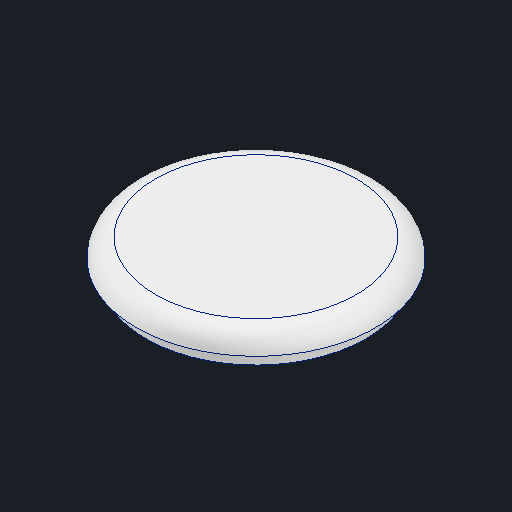
# Autodesk Inventor part: Tapa
Saved by Autodesk Inventor 2025.3 (Build 293356030, 356C)
## iProperties
Created: 2024-12-23
Part Number: Tapa
Material: Aluminio 6061
Document SubType Name: Modeling
Designer: Usuario
Density: 2.7 g/cm^3
Appearance: Aluminio - Plano
Mass: 96.7212 g
Surface Area: 197.809 cm^2
Volume: 96.7212 cm^3
Author: Usuario
Autodesk Inventor part; units mm, degrees
ref_plane "YZ Plane" through (0, 0, 0) normal (1, 0, 0) x (0, 1, 0)
ref_plane "XZ Plane" through (0, 0, 0) normal (0, 1, 0) x (-1, 0, 0)
ref_plane "XY Plane" through (0, 0, 0) normal (0, 0, 1) x (1, 0, 0)
sketch "Boceto1" plane through (0, 0, 0) normal (0, 1, 0) x (-1, 0, 0)
  circle A0 centre (0, 0) radius 50
  dimension "Diametro" = 100
  constraints: 1 centre point, 1 coincident
  measures "Diametro" diameter of A0
extrude "Extrusión1" add sketch "Boceto1" against normal blind 8
fillet "Empalme1" radius 8 1 edges at (50, 0, 0)
sketch "Boceto2" plane through (0, -8, 0) normal (0, -1, 0) x (1, 0, 0)
  circle A0 centre (0, 0) radius 46
  circle A1 centre (0, 0) radius 50 projected
  dimension "d22" = 4
  constraints: 1 centre point, 1 coincident
  measures "d22" radial gap between concentric circles of A1 A0
extrude "Extrusión3" add sketch "Boceto2" along normal blind 6 contours A0
sketch "Boceto3" plane through (0, -14, 0) normal (0, -1, 0) x (1, 0, 0)
  circle A0 centre (0, 0) radius 9
  point P0 (-37.5, 0)
  point P1 (-18.75, -32.476)
  point P2 (18.75, -32.476)
  point P3 (37.5, 0)
  point P4 (18.75, 32.476)
  point P5 (-18.75, 32.476)
  dimension "d25" = 37.5
  dimension "d35" = 360
  dimension "d37" = 18
  constraints: 1 centre point, 1 coincident, 1 horizontal alignment, 7 other
  measures "d25" distance of point (0, 0) point (-37.5, 0)
  measures "d37" diameter of A0
hole "Agujero2" at (-37.5, -14, 0) at (-18.75, -14, 32.476) at (-18.75, -14, -32.476) at (18.75, -14, 32.476) at (37.5, -14, 0) at (18.75, -14, -32.476) direction (0, 1, 0) diameter 2.459 depth 8.8 thread size "M3x0.5" class "6H" standard "ANSI Metric M Profile"
extrude "Extrusión4" cut sketch "Boceto3" against normal blind 5
